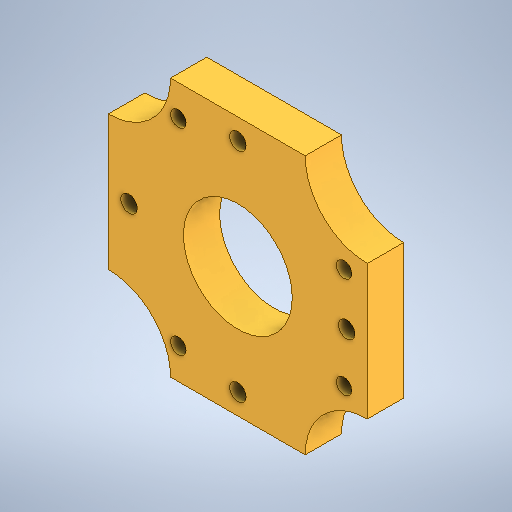
# Autodesk Inventor part: CONECTOR DE ACOPLE A AVION
Saved by Autodesk Inventor 2025.3 (Build 293356030, 356C)
## iProperties
Created: 2025-07-11
Part Number: CONECTOR DE ACOPLE A AVION
Material: Generic
Document SubType Name: Modeling
Designer: jv
Density: 1 g/cm^3
Appearance: Default(1)
Author: jv
Autodesk Inventor part; units mm, degrees
ref_plane "YZ Plane" through (0, 0, 0) normal (1, 0, 0) x (0, 1, 0)
ref_plane "XZ Plane" through (0, 0, 0) normal (0, 1, 0) x (-1, 0, 0)
ref_plane "XY Plane" through (0, 0, 0) normal (0, 0, 1) x (1, 0, 0)
sketch "Sketch1" plane through (0, 0, 0) normal (0, 0, 1) x (1, 0, 0)
  line L0 (-25, 25) -> (25, 25)
  line L1 (25, 25) -> (25, -25)
  line L2 (25, -25) -> (-25, -25)
  line L3 (-25, -25) -> (-25, 25)
  circle A0 centre (0, 0) radius 10.5
  circle A1 centre (-11.5, 19) radius 1.5
  circle A2 centre (20.5, 9.75) radius 1.5
  line L4 (20.5, 0) -> (20.5, 9.75)
  line L5 (-53.0419, 0) -> (53.0419, 0)
  circle A3 centre (20.5, -9.75) radius 1.5
  circle A4 centre (-11.5, -19) radius 1.5
  point P0 (0, 25)
  point P1 (25, 0)
  point P2 (25, 9.75)
  point P3 (22, 9.75)
  point P4 (-10, 19)
  point P5 (20.5, 11.25)
  point P6 (20.5, -11.25)
  point P7 (-11.5, 20.5)
  point P8 (-11.5, -20.5)
  dimension "d49" = 3
  dimension "d56" = 30.3101
  dimension "d0" = 50
  dimension "d1" = 21
  dimension "d2" = 50
  dimension "d3" = 3
  dimension "d6" = 3
  dimension "d10" = 19.5
  dimension "d11" = 11.5
  dimension "d12" = 20.5
  dimension "d46" = 13.5
  dimension "d48" = 10.7005
  dimension "d50" = 10.7005
  dimension "d52" = 35
  dimension "d53" = 38
  dimension "d54" = 16.5
  dimension "d55" = 10.2092
  dimension "d60" = 40.0182
  dimension "d61" = 35
  dimension "d62" = 22.5
  dimension "d63" = 41
  dimension "d64" = 3
  constraints: 12 end point, 7 vertical alignment, 4 horizontal alignment, 4 point on circle, 3 centre point, 3 midpoint, 2 coincident, 2 horizontal, 2 parallel, 2 symmetric about line, 1 perpendicular, 1 point on line, 1 vertical, 6 other
  measures "d0" distance of L0.start L0.end
  measures "d1" diameter of A0
  measures "d2" distance of L2.end L0.start
  measures "d3" diameter of A1
  measures "d6" diameter of A2
  measures "d10" diameter of L4.end L5
  measures "d11" horizontal distance of point (0, 0) A1.centre
  measures "d12" horizontal distance of point (0, 0) L4.end
  measures "d46" distance from line of L3 A1.centre
  measures "d53" distance of point (-11.5, -19) A1.centre
  measures "d61" distance from line of L1 A1.start
  measures "d62" distance of A2.end point (20.5, -11.25)
  measures "d63" distance of A1.end point (-11.5, -20.5)
  measures "d64" distance from line of L1 A2.start
extrude "Extrusion1" add sketch "Sketch1" along normal blind 7 contours L0 L1 L5 A0 L3 | L5 A0 L1 L2 L3
sketch "Sketch3" plane through (0, 0, 7) normal (0, 0, 1) x (1, 0, 0)
  line L0 (-4, 25) -> (4, 25)
  line L1 (4, 25) -> (4, -25)
  line L2 (4, -25) -> (-4, -25)
  line L3 (-4, -25) -> (-4, 25)
  circle A0 centre (12.5, 0) radius 2
  circle A1 centre (-12.5, 0) radius 2
  circle A2 centre (21, 0) radius 1.6
  circle A3 centre (0, 21) radius 1.6
  circle A4 centre (-21, 0) radius 1.6
  circle A5 centre (0, -21) radius 1.6
  line L4 (-25, -4) -> (-25, 4)
  line L5 (-25, 4) -> (25, 4)
  line L6 (25, -4) -> (-25, -4)
  line L7 (25, 4) -> (25, -4)
  circle A6 centre (0, 21) radius 4
  circle A7 centre (21, 0) radius 4
  circle A8 centre (-21, 0) radius 4
  circle A9 centre (0, -21) radius 4
  circle A10 centre (12.5, 12.5) radius 8.5
  circle A11 centre (-12.5, 12.5) radius 8.5
  circle A12 centre (-12.5, -12.5) radius 8.5
  circle A13 centre (12.5, -12.5) radius 8.5
  circle A14 centre (0, 0) radius 4
  circle A15 centre (0, 9.5) radius 2
  circle A16 centre (0, -9.5) radius 2
  point P0 (4, 0)
  point P1 (0, 25)
  point P2 (-25, 0)
  point P3 (0, 4)
  dimension "d75" = 4
  dimension "d76" = 360
  dimension "d77" = 3.2
  dimension "d78" = 360
  dimension "d79" = 8
  dimension "d80" = 90
  dimension "d81" = 50
  dimension "d82" = 42
  dimension "d83" = 4
  dimension "d84" = 17
  dimension "d85" = 360
  dimension "d86" = 4
  dimension "d87" = 360
  dimension "d88" = 19
  dimension "d89" = 25
  constraints: 16 end point, 14 centre point, 6 coincident, 3 horizontal alignment, 2 midpoint, 2 parallel, 2 tangent, 2 vertical alignment, 1 horizontal, 1 perpendicular, 45 other
  measures "d75" diameter of A0
  measures "d77" diameter of A2
  measures "d79" distance of L1.end L3.start
  measures "d81" distance between parallel lines of L2 L0
  measures "d82" distance of A5.centre A3.centre
  measures "d83" distance of point (0, 25) point (0, 21)
  measures "d84" diameter of A10
  measures "d86" diameter of A15
  measures "d88" distance of A16.centre A15.centre
  measures "d89" distance of A0.centre A1.centre
extrude "Extrusion3" cut sketch "Sketch3" against normal blind 7 contours A2 | A3 | A4 | A5
fillet "Fillet1" radius 12 4 edges at (-25, 25, 3.5) (25, 25, 3.5) (25, -25, 3.5) (-25, -25, 3.5) inverted yes
body "Solid1"
